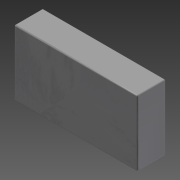
# Autodesk Inventor part: PSUUltibots
Saved by Autodesk Inventor 2016 (Build 200138000, 138)
## iProperties
Category: Electronics
Created: 2014-02-17
Part Number: PSUUltibots
Material: Generic
Document SubType Name: Modeling
Designer: Jack
Density: 1 g/cm^3
Appearance: Default
Mass: 1110.08 g
Surface Area: 846.592 cm^2
Volume: 1110.08 cm^3
Vendor: MakersToolWorks
Author: Jack
Title: PSU
Autodesk Inventor part; units mm, degrees
ref_plane "YZ Plane" through (0, 0, 0) normal (1, 0, 0) x (0, 1, 0)
ref_plane "XZ Plane" through (0, 0, 0) normal (0, 1, 0) x (-1, 0, 0)
ref_plane "XY Plane" through (0, 0, 0) normal (0, 0, 1) x (1, 0, 0)
sketch "Sketch1" plane through (0, 0, 0) normal (0, 1, 0) x (-1, 0, 0)
  line L0 (0, 0) -> (215, 0)
  line L1 (215, 0) -> (215, 115)
  line L2 (215, 115) -> (0, 115)
  line L3 (0, 115) -> (0, 0)
  dimension "d0" = 215
  dimension "d1" = 115
  constraints: 8 end point, 2 perpendicular, 1 horizontal, 1 parallel
  measures "d0" distance of L0.start L0.end
  measures "d1" distance of L0.end L1.end
extrude "Extrusion1" add sketch "Sketch1" along normal blind 50
sketch "Sketch2" plane through (0, 50, 0) normal (0, 1, 0) x (1, 0, 0)
  line L0 (0, 0) -> (-215, 0) projected
  line L1 (-215, 0) -> (-215, -115) projected
  line L2 (-215, -115) -> (0, -115) projected
  line L3 (0, -115) -> (0, 0) projected
  line L4 (-215, -3) -> (-187.5, -3)
  line L5 (-187.5, -3) -> (-187.5, -112)
  line L6 (-187.5, -112) -> (-215, -112)
  dimension "d4" = 27.5
  dimension "d5" = 3
  dimension "d6" = 3
  constraints: 6 end point, 3 perpendicular, 2 point on line
  measures "d4" distance of L4.start L4.end
  measures "d5" distance between parallel lines of L2 L6
  measures "d6" distance between parallel lines of L0 L4
extrude "Extrusion2" cut sketch "Sketch2" against normal blind 45 contours L4 L5 L6 L1
fillet "Fillet1" radius 2 10 edges at (-107.5, 50, 115) (-107.5, 0, 115) (-107.5, 50, 0) (0, 50, 57.5) (0, 0, 57.5) (0, 25, 115) (0, 25, 0) (-215, 25, 115) (-215, 0, 57.5) (-215, 25, 0)
fillet "Fillet2" radius 2 1 edges at (-187.5, 50, 57.5)
sketch "Sketch3" plane through (0, 5, 0) normal (0, 1, 0) x (1, 0, 0)
  line L0 (-215, -112) -> (-215, -3) projected
  line L1 (-187.5, -112) -> (-215, -112) projected
  line L2 (-187.5, -3) -> (-187.5, -112) projected
  line L3 (-215, -3) -> (-187.5, -3) projected
  line L4 (-212, -110) -> (-212, -38)
  line L5 (-212, -38) -> (-187.5, -38)
  line L6 (-212, -110) -> (-187.5, -110)
  point P0 (0, 0)
  dimension "d14" = 3
  dimension "d15" = 2
  dimension "d16" = 72
  constraints: 6 end point, 2 perpendicular, 2 point on line, 1 parallel
  measures "d14" distance between parallel lines of L0 L4
  measures "d15" distance between parallel lines of L1 L6
  measures "d16" distance of L4.start L4.end
extrude "Extrusion3" add sketch "Sketch3" along normal blind 5 contours L6 L4 L5 L2
sketch "Sketch4" plane through (0, 10, 0) normal (0, 1, 0) x (1, 0, 0)
  line L0 (-212, -110) -> (-187.5, -110) projected
  line L1 (-212, -38) -> (-212, -110) projected
  circle A0 centre (-206, -45.5) radius 3
  circle A1 centre (-206, -55) radius 3
  circle A2 centre (-206, -64.5) radius 3
  circle A3 centre (-206, -74) radius 3
  circle A4 centre (-206, -83.5) radius 3
  circle A5 centre (-206, -93) radius 3
  circle A6 centre (-206, -102.5) radius 3
  point P0 (0, 0)
  dimension "d19" = 6
  dimension "d25" = 9.5
  dimension "d26" = 9.5
  dimension "d27" = 9.5
  dimension "d28" = 9.5
  dimension "d29" = 9.5
  dimension "d30" = 9.5
  dimension "d31" = 7.5
  dimension "d32" = 6
  constraints: 7 centre point, 6 equal radius, 6 vertical alignment
  measures "d19" diameter of A0
  measures "d25" distance of A1.centre A0.centre
  measures "d26" distance of A6.centre A5.centre
  measures "d27" distance of A5.centre A4.centre
  measures "d28" distance of A4.centre A3.centre
  measures "d29" distance of A3.centre A2.centre
  measures "d30" distance of A2.centre A1.centre
  measures "d31" distance from line of L0 A6.centre
  measures "d32" distance from line of L1 A0.centre
extrude "Extrusion4" add sketch "Sketch4" along normal blind 6
fillet "Fillet3" radius 2 3 edges at (-214.4142, 0.5858, 0.5858) (-0.5858, 0.5858, 0.5858) (-107.5, 0, 0)
body "Solid1"
